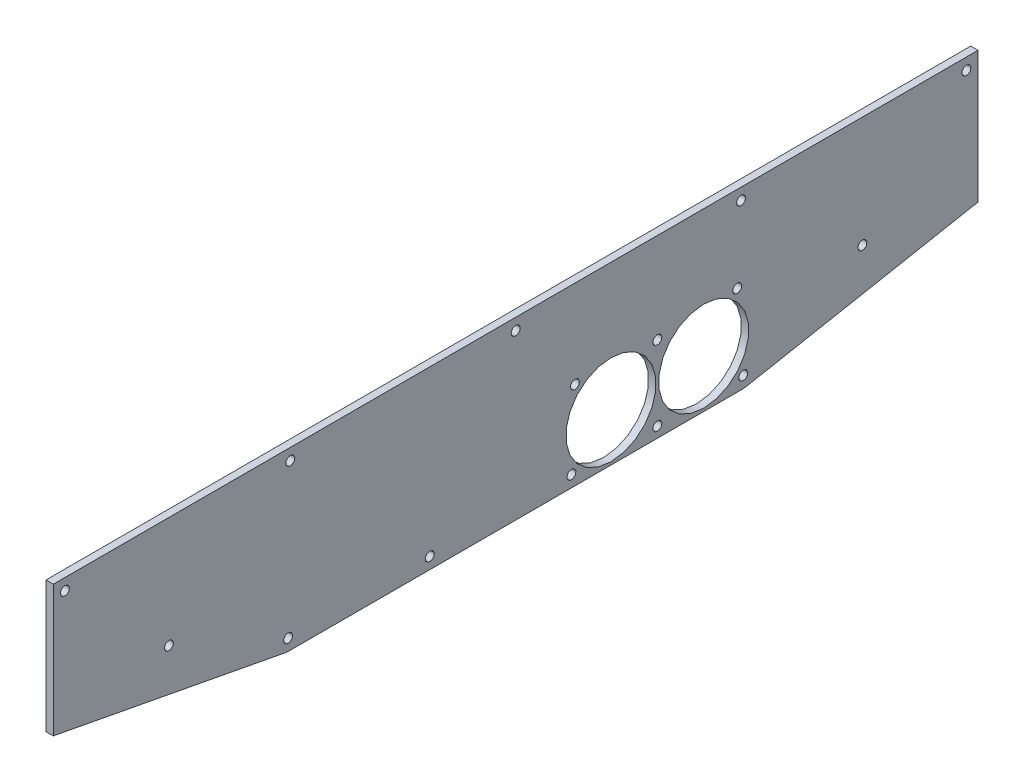
# Autodesk Inventor part: InsideChassiPlate3.0
Saved by Autodesk Inventor 2023 (Build 270158000, 158)
## iProperties
Created: 2022-09-18
Part Number: InsideChassiPlate3.0
Material: Generic
Document SubType Name: Modeling
Designer: deli
Density: 1 g/cm^3
Appearance: Default
Author: deli
Autodesk Inventor part; units mm, degrees
ref_plane "YZ Plane" through (0, 0, 0) normal (1, 0, 0) x (0, 1, 0)
ref_plane "XZ Plane" through (0, 0, 0) normal (0, 1, 0) x (-1, 0, 0)
ref_plane "XY Plane" through (0, 0, 0) normal (0, 0, 1) x (1, 0, 0)
sketch "Sketch1" plane through (0, 0, 0) normal (1, 0, 0) x (0, 1, 0)
  line L0 (166.4208, 143.2964) -> (147.3544, 42.6727) projected
  arc A0 (147.3544, 42.6727) -> (147.267, 41.7418) centre (152.267, 41.7418) ccw projected
  line L1 (147.267, 41.7418) -> (147.267, -155.149) projected
  arc A1 (147.267, -155.149) -> (147.3544, -156.0799) centre (152.267, -155.149) ccw projected
  line L2 (147.3544, -156.0799) -> (166.4208, -256.7036) projected
  line L3 (166.4208, -256.7036) -> (253.267, -256.7036) projected
  line L4 (253.267, -256.7036) -> (253.267, 143.2964) construction
  line L5 (253.267, 143.2964) -> (166.4208, 143.2964) projected
  circle A2 centre (152.267, -19.538) radius 2 projected
  circle A3 centre (218.267, 40.7964) radius 2 projected
  circle A4 centre (218.267, -154.2036) radius 2 projected
  circle A5 centre (218.267, -251.7036) radius 2 projected
  circle A6 centre (186.186, -152.5532) radius 2 projected
  circle A7 centre (152.267, -80.8178) radius 2 projected
  circle A8 centre (151.8757, -117.9834) radius 2 projected
  circle A9 centre (184.1582, -117.9834) radius 2 projected
  circle A10 centre (168.017, -138.0464) radius 7 construction
  circle A11 centre (168.017, -97.9204) radius 7 construction
  circle A12 centre (175.267, -206.7036) radius 2 projected
  circle A13 centre (175.267, 93.2964) radius 2 projected
  circle A14 centre (218.267, 138.2964) radius 2 projected
  circle A15 centre (185.2844, -82.3513) radius 2 projected
  circle A16 centre (218.267, -56.7036) radius 2 projected
  circle A17 centre (152.267, 41.7418) radius 2 projected
  circle A18 centre (152.267, -155.149) radius 2 projected
  circle A19 centre (168.017, -97.9204) radius 19.5
  circle A20 centre (168.017, -138.0464) radius 19.5
  circle A21 centre (137.7375, -163.4822) radius 7 construction
  circle A22 centre (137.7375, -203.6081) radius 7 construction
  line L6 (223.267, 143.2964) -> (223.267, -256.7036)
  point P0 (0, 0)
  dimension "d0" = 39
  dimension "d1" = 39
  dimension "d2" = 5
  constraints: 2 centre point, 2 coincident, 2 end point, 2 point on line, 1 perpendicular
  measures "d0" diameter of A19
  measures "d1" diameter of A20
  measures "d2" distance from line of L6 A14.centre
extrude "Extrusion1" add sketch "Sketch1" along normal blind 3.175
equation "\"d1\" = d0"
body "Solid1"
